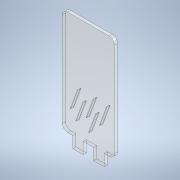
# Autodesk Inventor part: Scheibe
Saved by Autodesk Inventor 2021 (Build 250183000, 183)
## iProperties
Created: 2021-03-05
Part Number: Scheibe
Material: Glas
Document SubType Name: Modeling
Designer: Tilman
Density: 2.18 g/cm^3
Appearance: Klar
Author: Tilman
Autodesk Inventor part; units mm, degrees
ref_plane "YZ Plane" through (0, 0, 0) normal (1, 0, 0) x (0, 1, 0)
ref_plane "XZ Plane" through (0, 0, 0) normal (0, 1, 0) x (-1, 0, 0)
ref_plane "XY Plane" through (0, 0, 0) normal (0, 0, 1) x (1, 0, 0)
sketch "Skizze1" plane through (0, 0, 0) normal (0, 0, 1) x (1, 0, 0)
  line L0 (0, 5) -> (0, 95)
  line L1 (5, 100) -> (45, 100)
  line L2 (50, 95) -> (50, 5)
  arc A0 (5, 100) -> (0, 95) centre (5, 95) ccw
  arc A1 (50, 95) -> (45, 100) centre (45, 95) ccw
  arc A2 (45, 0) -> (50, 5) centre (45, 5) ccw
  arc A3 (0, 5) -> (5, 0) centre (5, 5) ccw
  line L3 (10, 0) -> (10, -11)
  line L4 (10, -11) -> (20, -11)
  line L5 (20, -11) -> (20, 0)
  line L6 (30, 0) -> (30, -11)
  line L7 (30, -11) -> (40, -11)
  line L8 (40, -11) -> (40, 0)
  line L9 (5, 0) -> (10, 0)
  line L10 (20, 0) -> (30, 0)
  line L11 (40, 0) -> (45, 0)
  line L12 (14.3404, 40) -> (14.8102, 39.829)
  line L13 (14.8102, 39.829) -> (7.9698, 21.0351)
  line L14 (7.9698, 21.0351) -> (7.5, 21.2061)
  line L15 (7.5, 21.2061) -> (14.3404, 40)
  line L16 (19.6299, 32.4397) -> (20.0998, 32.2687)
  line L17 (20.0998, 32.2687) -> (13.2594, 13.4748)
  line L18 (13.2594, 13.4748) -> (12.7895, 13.6459)
  line L19 (12.7895, 13.6459) -> (19.6299, 32.4397)
  line L20 (29.5432, 40) -> (30.013, 39.829)
  line L21 (30.013, 39.829) -> (23.1726, 21.0351)
  line L22 (22.7028, 21.2061) -> (29.5432, 40)
  line L23 (23.1726, 21.0351) -> (22.7028, 21.2061)
  line L24 (42.3412, 40) -> (42.8111, 39.829)
  line L25 (35.5008, 21.2061) -> (42.3412, 40)
  line L26 (42.8111, 39.829) -> (35.9707, 21.0351)
  line L27 (35.9707, 21.0351) -> (35.5008, 21.2061)
  line L28 (31.9383, 28.9336) -> (32.4081, 28.7626)
  line L29 (25.0979, 10.1397) -> (31.9383, 28.9336)
  line L30 (32.4081, 28.7626) -> (25.5677, 9.9687)
  line L31 (25.5677, 9.9687) -> (25.0979, 10.1397)
  point P0 (0, 0)
  dimension "d1" = 50
  dimension "d3" = 5
  dimension "d4" = 11
  dimension "d5" = 10
  dimension "d6" = 100
  dimension "d9" = 0.5
  dimension "d10" = 20
  dimension "d11" = 20
  dimension "d12" = 7.5
  dimension "d14" = 40
  constraints: 64 end point, 16 parallel, 13 equal length, 8 point on circle, 7 tangent, 6 perpendicular, 5 horizontal alignment, 4 centre point, 4 horizontal, 3 equal radius, 3 vertical, 2 collinear, 1 vertical alignment
  measures "d1" distance between parallel lines of L2 L0
  measures "d3" radius of A0
  measures "d4" distance of L3.start L3.end
  measures "d5" distance of L3.end L4.end
  measures "d6" distance between parallel lines of L10 L1
  measures "d9" distance of L12.start L12.end
  measures "d10" distance of L12.end L13.end
  measures "d11" angle of L0 L15
  measures "d12" distance from line of L0 L14.end
  measures "d14" distance from line of L9 L12.start
extrude "Extrusion1" add sketch "Skizze1" along normal blind 3
